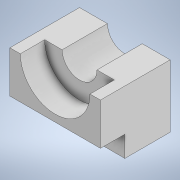
# Autodesk Inventor part: 2-4
Saved by Autodesk Inventor 2020 (Build 240168000, 168)
## iProperties
Created: 2023-11-21
Part Number: 2-4
Material: 常规
Document SubType Name: Modeling
Designer: Z
Density: 1 g/cm^3
Appearance: 默认
Author: Z
Autodesk Inventor part; units mm, degrees
ref_plane "YZ Plane" through (0, 0, 0) normal (1, 0, 0) x (0, 1, 0)
ref_plane "XZ Plane" through (0, 0, 0) normal (0, 1, 0) x (-1, 0, 0)
ref_plane "XY Plane" through (0, 0, 0) normal (0, 0, 1) x (1, 0, 0)
sketch "草图1" plane through (0, 0, 0) normal (0, 0, 1) x (1, 0, 0)
  line L0 (-13, 9) -> (13, 9)
  line L1 (13, 9) -> (13, -9)
  line L2 (13, -9) -> (-13, -9)
  line L3 (-13, -9) -> (-13, 9)
  line L4 (-13, 9) -> (13, -9) construction
  line L5 (13, 9) -> (-13, -9) construction
  point P0 (0, 0)
  dimension "d0" = 26
  dimension "d1" = 18
  constraints: 12 end point, 2 midpoint, 2 parallel, 1 horizontal, 1 perpendicular
  measures "d0" distance of L1.end L2.end
  measures "d1" distance of L0.end L1.end
extrude "拉伸1" add sketch "草图1" along normal blind 13
sketch "草图2" plane through (0, 0, 13) normal (0, 0, 1) x (1, 0, 0)
  line L0 (13, 9) -> (-13, 9) projected
  line L1 (13, -9) -> (13, 9) projected
  line L2 (-13, 9) -> (13, 9)
  line L3 (13, 9) -> (13, -3)
  line L4 (13, -3) -> (-13, -3)
  line L5 (-13, -3) -> (-13, 9)
  arc A0 (-10, 9) -> (10, 9) centre (0, 9) ccw
  point P0 (0, 0)
  point P1 (10, 9)
  dimension "d4" = 12
  dimension "d5" = 20
  constraints: 8 end point, 3 point on line, 2 parallel, 2 point on circle, 1 centre point, 1 horizontal, 1 midpoint, 1 perpendicular
  measures "d4" distance of L2.end L3.end
  measures "d5" diameter of A0
extrude "拉伸2" add sketch "草图2" along normal blind 7 contours L1 L4 L5 L0 A0
sketch "草图3" plane through (0, 0, 13) normal (0, 0, 1) x (1, 0, 0)
  line L0 (10, 9) -> (-10, 9) projected
  arc A0 (-5, 9) -> (5, 9) centre (0, 9) ccw
  point P0 (0, 0)
  dimension "d8" = 10
  constraints: 2 point on circle, 2 point on line, 1 centre point, 1 midpoint
  measures "d8" diameter of A0
extrude "拉伸3" cut sketch "草图3" against normal blind 13
